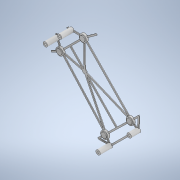
# Autodesk Inventor part: print006_Grundform_Boden
Saved by Autodesk Inventor 2020.3 (Build 243373000, 373)
## iProperties
Created: 2020-03-04
Part Number: print006_Grundform_Boden
Material: Generic
Document SubType Name: Modeling
Designer: Mara
Density: 1 g/cm^3
Appearance: Default
d0: 2,000 mm
d2: 1,000 mm
d3: 5,563 mm
d8: 5,563 mm
d9: 2,000 mm
d10: 170,74 deg
d11: 2,000 mm
d12: 163,54 deg
d21: 60,427 mm
d22: 66,844 mm
d24: 47,207 mm
d25: 2,000 mm
d26: 2,000 mm
d27: 81,43 deg
d28: 93,01 deg
d29: 53,219 mm
d30: 2,000 mm
d31: 2,000 mm
d32: 2,000 mm
d33: 2,000 mm
d34: 2,000 mm
d35: 2,000 mm
d36: 66,67 deg
d37: 45,78 deg
d39: 92,41 deg
d40: 87,65 deg
d42: 89,80 deg
d45: 1,000 mm
d46: 18,000 mm
d48: 2,000 mm
d49: 6,361 mm
d51: 27,126 mm
d52: 44,927 mm
d53: 48,903 mm
d54: 29,968 mm
d55: 20,958 mm
d56: 2,000 mm
d57: 2,000 mm
d58: 2,000 mm
d59: 64,660 mm
d60: 67,034 mm
d61: 34,990 mm
d62: 27,853 mm
d63: 15,000 mm
d64: 11,000 mm
d65: 20,850 mm
d66: 17,000 mm
d67: 11,000 mm
d70: 10,300 mm
d71: 3,845 mm
d72: 5,442 mm
d73: 5,436 mm
d75: 5,541 mm
d76: 5,457 mm
d77: 3,113 mm
d78: 2,630 mm
d80: 3,207 mm
d82: 5,463 mm
d87: 1,000 mm
d88: 0,00 deg
d93: 1,000 mm
d94: 4,757 mm
d95: 1,000 mm
d96: 4,757 mm
d99: 1,000 mm
d100: 4,757 mm
d105: 17,500 mm
d106: 1,000 mm
d107: 0,00 deg
d108: 0,00 deg
d109: 4,757 mm
d110: 1,000 mm
d111: 13,000 mm
d112: 1,000 mm
d113: 0,00 deg
d114: 0,00 deg
d115: 2,049 mm
d116: 2,049 mm
d117: 2,049 mm
d118: 3,300 mm
d119: 0,00 deg
d120: 2,049 mm
d121: 3,300 mm
d122: 0,00 deg
d123: 2,000 mm
d124: 0,00 deg
d125: 2,000 mm
d127: 2,000 mm
d128: 1,000 mm
d129: 0,00 deg
d130: 2,000 mm
d131: 2,000 mm
d134: 2,000 mm
d135: 2,000 mm
Author: Mara
Autodesk Inventor part; units mm, degrees
ref_plane "YZ Plane" through (0, 0, 0) normal (1, 0, 0) x (0, 1, 0)
ref_plane "XZ Plane" through (0, 0, 0) normal (0, 1, 0) x (-1, 0, 0)
ref_plane "XY Plane" through (0, 0, 0) normal (0, 0, 1) x (1, 0, 0)
sketch "Sketch1" plane through (0, 0, 0) normal (0, 0, 1) x (1, 0, 0)
  line L0 (-49.2977, 34.5359) -> (-22.38, 61.3045)
  line L1 (-47.8874, 33.1177) -> (-20.9698, 59.8864)
  line L2 (-49.2977, 34.5359) -> (-47.8874, 33.1177) construction
  circle A0 centre (-52.4729, 29.968) radius 5.563
  circle A1 centre (-17.7815, 64.4351) radius 5.563
  line L3 (-13.9364, 68.4553) -> (-0.1095, 78.3456)
  line L4 (-12.7631, 66.8356) -> (1.0638, 76.7259)
  line L5 (-57.711, 28.0946) -> (-67.3885, 22.8653)
  line L6 (-56.7093, 26.3625) -> (-66.3869, 21.1332)
  line L7 (-49.5894, 25.2106) -> (10.1162, -41.4966)
  circle A2 centre (14.4958, -44.9268) radius 5.563
  circle A3 centre (52.6405, -7.8239) radius 5.563
  line L8 (-48.0932, 26.5378) -> (11.6124, -40.1694)
  line L9 (-14.6001, 59.8716) -> (48.0505, -4.6808)
  line L10 (-13.1915, 61.292) -> (49.4591, -3.2604)
  line L11 (49.4227, -12.3618) -> (19.1106, -41.8201)
  line L12 (48.0258, -10.9306) -> (17.7136, -40.3888)
  line L13 (11.2885, -49.4721) -> (3.9093, -56.6581)
  line L14 (9.8883, -48.0441) -> (2.5091, -55.23)
  line L15 (57.2511, -4.7111) -> (65.1179, 2.9774)
  line L16 (55.8523, -3.2817) -> (63.7191, 4.4068)
  line L17 (-39.0119, 41.9442) -> (29.6903, -28.7495)
  line L18 (-37.5936, 43.3546) -> (31.1246, -27.3556)
  line L19 (-55.5021, 34.6339) -> (-60.6997, 47.8234)
  line L20 (-53.6558, 35.4038) -> (-59.1552, 49.3593)
  line L21 (-23.223, 65.5915) -> (-42.1516, 65.9031)
  line L22 (-23.2803, 63.5921) -> (-44.1303, 63.9354)
  circle A4 centre (-17.2221, 20.9576) radius 3.1804
  line L23 (13.0651, -39.5509) -> (-14.9644, 18.7175)
  line L24 (11.2563, -40.4044) -> (-16.7485, 17.8127)
  line L25 (-14.0533, 20.686) -> (47.9022, -4.9092)
  line L26 (-14.8421, 18.848) -> (47.1775, -6.7738)
  line L27 (-18.703, 58.9489) -> (-18.2564, 23.9652)
  line L28 (-16.7032, 58.9776) -> (-16.2565, 23.9879)
  line L29 (-47.4654, 27.5447) -> (-20.389, 20.6653)
  line L30 (-46.932, 29.4728) -> (-19.9371, 22.614)
  line L31 (-0.1095, 78.3456) -> (1.0638, 76.7259)
  line L32 (-44.073, 65.9347) -> (-44.1303, 63.9354) construction
  line L33 (-59.1552, 49.3593) -> (-61.0015, 48.5894) construction
  line L34 (-67.3885, 22.8653) -> (-66.3869, 21.1332)
  line L35 (3.9093, -56.6581) -> (2.5091, -55.23)
  line L36 (65.1179, 2.9774) -> (63.7191, 4.4068)
  line L37 (-59.1552, 49.3593) -> (-60.6997, 47.8234)
  line L38 (-44.1303, 63.9354) -> (-42.1516, 65.9031)
  line L39 (-42.1516, 65.9031) -> (-44.073, 65.9347) construction
  line L40 (-60.6997, 47.8234) -> (-61.0015, 48.5894) construction
  point P0 (0, 0)
  point P1 (9.143, -43.4122)
  point P2 (-19.963, 60.8956)
  point P3 (18.6755, -41.2556)
  point P4 (19.8991, -43.603)
  point P5 (47.2964, -9.3692)
  point P6 (58.0343, -9.1855)
  point P7 (55.8444, -3.2761)
  point P8 (16.2732, -50.1982)
  point P9 (18.0227, -49.2289)
  point P10 (56.2951, -12.0181)
  point P11 (57.5423, -10.4544)
  point P12 (-20.321, 22.7115)
  point P13 (-20.9757, 59.8805)
  point P14 (-18.6091, 23.8197)
  point P15 (10.5981, -39.0362)
  point P16 (31.0842, -30.1838)
  point P17 (32.5185, -28.7899)
  point P18 (31.1246, -27.3556)
  point P19 (-13.0632, 18.1131)
  point P20 (-13.5186, 15.7119)
  point P21 (29.6903, -28.7495)
  point P22 (-20.0433, 22.4258)
  dimension "d49" = 6.3609
  dimension "d0" = 2
  dimension "d2" = 1
  dimension "d3" = 5.563
  dimension "d8" = 5.563
  dimension "d9" = 2
  dimension "d10" = 170.735
  dimension "d11" = 2
  dimension "d12" = 163.544
  dimension "d21" = 60.4275
  dimension "d22" = 66.8436
  dimension "d24" = 47.2075
  dimension "d25" = 2
  dimension "d26" = 2
  dimension "d27" = 81.433
  dimension "d28" = 93.011
  dimension "d29" = 53.2188
  dimension "d30" = 2
  dimension "d31" = 2
  dimension "d32" = 2
  dimension "d33" = 2
  dimension "d34" = 2
  dimension "d35" = 2
  dimension "d36" = 66.667
  dimension "d37" = 45.784
  dimension "d39" = 92.41
  dimension "d40" = 87.648
  dimension "d42" = 89.8
  dimension "d45" = 1
  dimension "d46" = 18
  dimension "d48" = 2
  dimension "d51" = 27.126
  dimension "d52" = 44.9268
  dimension "d53" = 48.9027
  dimension "d54" = 29.968
  dimension "d55" = 20.9576
  dimension "d56" = 2
  dimension "d57" = 2
  dimension "d58" = 2
  dimension "d59" = 64.6596
  dimension "d60" = 67.0343
  dimension "d61" = 34.9897
  dimension "d62" = 27.8525
  dimension "d63" = 15
  dimension "d64" = 11
  dimension "d65" = 20.85
  dimension "d66" = 17
  dimension "d67" = 11
  dimension "d70" = 10.3
  dimension "d71" = 3.8451
  dimension "d72" = 5.4415
  dimension "d73" = 5.4358
  dimension "d75" = 5.5409
  dimension "d76" = 5.4575
  dimension "d77" = 3.1128
  dimension "d78" = 2.6305
  dimension "d80" = 3.2073
  dimension "d82" = 5.463
  constraints: 83 end point, 27 parallel, 4 point on line, 2 perpendicular, 62 other
  measures "d0" distance between parallel lines of L1 L0
  measures "d2" distance from line of L0 point (-52.473, 29.968)
  measures "d3" distance of L0.start point (-52.473, 29.968)
  measures "d8" distance of L0.end point (-17.782, 64.435)
  measures "d9" distance between parallel lines of L4 L3
  measures "d10" angle of L3 L0
  measures "d11" distance between parallel lines of L6 L5
  measures "d12" angle of L1 L6
  measures "d21" distance of point (-52.473, 29.968) point (0, 0)
  measures "d22" distance of point (0, 0) point (-17.782, 64.435)
  measures "d24" distance of point (0, 0) point (14.496, -44.927)
  measures "d25" distance between parallel lines of L7 L8
  measures "d26" distance between parallel lines of L9 L10
  measures "d27" angle of L10 L4
  measures "d28" angle of L8 L1
  measures "d29" distance of point (0, 0) point (52.641, -7.824)
  measures "d30" distance between parallel lines of L11 L12
  measures "d31" distance between parallel lines of L13 L14
  measures "d32" distance between parallel lines of L15 L16
  measures "d33" distance between parallel lines of L18 L17
  measures "d34" distance between parallel lines of L20 L19
  measures "d35" distance between parallel lines of L21 L22
  measures "d36" angle of L0 L20
  measures "d37" angle of L0 L22
  measures "d39" angle of L14 L7
  measures "d40" angle of L12 L8
  measures "d42" angle of L10 L16
  measures "d45" distance from line of point (-17.222, 20.958) L18
  measures "d46" distance from line of L17 point (-52.473, 29.968)
  measures "d48" distance between parallel lines of L23 L24
  measures "d51" distance of point (0, 0) point (-17.222, 20.958)
  measures "d52" vertical distance of point (0, 0) point (14.496, -44.927)
  measures "d53" distance of point (-52.473, 29.968) point (-17.782, 64.435)
  measures "d54" vertical distance of point (0, 0) point (-52.473, 29.968)
  measures "d55" vertical distance of point (-17.222, 20.958) point (0, 0)
  measures "d56" distance between parallel lines of L26 L25
  measures "d57" distance between parallel lines of L28 L27
  measures "d58" distance between parallel lines of L29 L30
  measures "d59" distance of L23.start L23.end
  measures "d60" distance of L25.start L25.end
  measures "d61" vertical distance of L28.start L28.end
  measures "d62" distance of L30.start L30.end
  measures "d63" distance of L20.start L20.end
  measures "d64" distance of L5.start L5.end
  measures "d65" horizontal distance of L22.start L22.end
  measures "d66" distance of L3.start L3.end
  measures "d67" distance of L15.start L15.end
  measures "d70" distance of L13.start L13.end
  measures "d71" horizontal distance of L3.start point (-17.782, 64.435)
  measures "d72" horizontal distance of point (-17.782, 64.435) L21.start
  measures "d73" vertical distance of point (-52.473, 29.968) L20.start
  measures "d75" horizontal distance of point (-52.473, 29.968) L30.start
  measures "d76" vertical distance of point (-17.782, 64.435) L28.start
  measures "d77" vertical distance of point (52.641, -7.824) L15.start
  measures "d78" vertical distance of point (52.641, -7.824) point (57.542, -10.454)
  measures "d80" horizontal distance of point (14.496, -44.927) L13.start
  measures "d82" horizontal distance of point (52.641, -7.824) L26.end
extrude "Extrusion3" add sketch "Sketch1" against normal blind 1 contours L0 A1 L1 A0 | A0 | A1 | A0 L19 L37 L20 | L22 L38 L21 A1 | L1 L18 A4 L30 L17 | A1 L28 A4 L27 | L17 A4 L29 A0 L30 | A0 L6 L34 L5 | L3 L31 L4 A1 | A4 L18 | L18 A4 L17 | L17 A4 | A4 L25 A3 L26 L18 | L18 L26 A4 | A1 L10 A3 L9 | A4 L23 L17 | L17 L23 A2 L8 L24 A4 | L8 L24 A2 L7 A0 | L18 L12 L17 L23 A4 L26 | A3 | L8 A2 L24 | A2 | L12 A3 L11 A2 | A2 L13 L35 L14 | L16 L36 L15 A3
sketch "Sketch3" plane through (0, 0, 0) normal (0, 0, 1) x (1, 0, 0)
  circle A0 centre (20.7546, -56.5669) radius 2.3783
  circle A1 centre (20.7546, -56.5669) radius 3.3783
  circle A2 centre (-36.8834, 64.7402) radius 2.3783
  circle A3 centre (-36.8834, 64.7402) radius 3.3783
  circle A4 centre (-58.3828, 44.2123) radius 2.3783
  circle A5 centre (-58.3828, 44.2123) radius 3.3783
  arc A6 (49.4227, -12.3618) -> (57.2511, -4.7111) centre (52.6405, -7.8239) ccw projected
  arc A7 (11.2885, -49.4721) -> (19.1106, -41.8201) centre (14.4958, -44.9268) ccw projected
  point P0 (0, 0)
  dimension "d93" = 1
  dimension "d94" = 4.7566
  dimension "d95" = 1
  dimension "d96" = 4.7566
  dimension "d99" = 1
  dimension "d100" = 4.7566
  constraints: 6 centre point, 3 coincident
  measures "d93" radial gap between concentric circles of A1 A0
  measures "d94" diameter of A0
  measures "d95" radial gap between concentric circles of A3 A2
  measures "d96" diameter of A2
  measures "d99" radial gap between concentric circles of A5 A4
  measures "d100" diameter of A4
extrude "Extrusion5" add sketch "Sketch3" along normal blind 17.5 and the other way blind 1
sketch "Sketch6" plane through (0, 0, 0) normal (0, 0, 1) x (1, 0, 0)
  circle A0 centre (62.8402, -15.6905) radius 2.3785
  circle A1 centre (62.8402, -15.6905) radius 3.3785
  point P0 (0, 0)
  dimension "d109" = 4.757
  dimension "d110" = 1
  constraints: 2 centre point, 1 coincident
  measures "d109" diameter of A0
  measures "d110" radial gap between concentric circles of A1 A0
extrude "Extrusion6" add sketch "Sketch6" along normal blind 13 and the other way blind 1
sketch "Sketch7" plane through (-58.3828, 44.2123, 17.5) normal (0, 0, 1) x (1, 0, 0)
  circle A0 centre (0, 0) radius 3.3783
  circle A1 centre (0, 0) radius 3.3783 projected
  circle A2 centre (0, 0) radius 1.3297
  circle A3 centre (21.4994, 20.5278) radius 3.3783
  circle A4 centre (21.4994, 20.5278) radius 3.3783 projected
  circle A5 centre (21.4994, 20.5278) radius 1.3293
  circle A6 centre (79.1375, -100.7793) radius 3.3783
  circle A7 centre (79.1375, -100.7793) radius 3.3783 projected
  circle A8 centre (79.1375, -100.7793) radius 1.3293
  point P0 (58.3828, -44.2123)
  dimension "d115" = 2.0486
  dimension "d116" = 2.049
  dimension "d117" = 2.049
  constraints: 6 centre point, 6 coincident, 3 concentric
  measures "d115" radial gap between concentric circles of A0 A2
  measures "d116" radial gap between concentric circles of A3 A5
  measures "d117" radial gap between concentric circles of A6 A8
extrude "Extrusion7" add sketch "Sketch7" against normal blind 3.3
sketch "Sketch8" plane through (62.8402, -15.6905, 13) normal (0, 0, 1) x (1, 0, 0)
  circle A0 centre (0, 0) radius 3.3785
  circle A1 centre (0, 0) radius 3.3785 projected
  circle A2 centre (0, 0) radius 1.3295
  point P0 (-62.8402, 15.6905)
  dimension "d120" = 2.049
  constraints: 2 centre point, 2 coincident, 1 concentric
  measures "d120" radial gap between concentric circles of A0 A2
extrude "Extrusion8" add sketch "Sketch8" against normal blind 3.3
sketch "Sketch9" plane through (0, 0, -1) normal (0, 0, -1) x (-1, 0, 0)
  circle A0 centre (58.3828, 44.2123) radius 2.3783
  arc A1 (58.0553, 46.568) -> (56.5363, 42.7134) centre (58.3828, 44.2123) ccw projected
  circle A2 centre (36.8834, 64.7402) radius 2.3783
  arc A3 (34.7075, 63.7802) -> (39.0899, 63.8524) centre (36.8834, 64.7402) ccw projected
  point P0 (0, 0)
  constraints: 2 centre point, 2 coincident, 2 concentric
extrude "Extrusion9" cut sketch "Sketch9" against normal blind 2
sketch "Sketch10" plane through (0, 0, 0) normal (0, 0, 1) x (1, 0, 0)
  arc A0 (49.4227, -12.3618) -> (57.2511, -4.7111) centre (52.6405, -7.8239) ccw projected
  line L0 (56.3201, -11.9961) -> (59.655, -14.5641)
  circle A1 centre (62.8402, -15.6905) radius 3.3785 projected
  line L1 (57.5579, -10.4251) -> (60.8502, -12.9602)
  arc A2 (11.2885, -49.4721) -> (19.1106, -41.8201) centre (14.4958, -44.9268) ccw projected
  line L2 (16.2829, -50.1949) -> (18.3621, -54.1818)
  circle A3 centre (20.7546, -56.5669) radius 3.3783 projected
  line L3 (18.0312, -49.2219) -> (20.1301, -53.2468)
  circle A4 centre (20.7546, -56.5669) radius 3.3783 projected
  arc A5 (11.2885, -49.4721) -> (19.1106, -41.8201) centre (14.4958, -44.9268) ccw projected
  line L4 (3.9093, -56.6581) -> (19.4284, -56.6581)
  circle A6 centre (20.7546, -56.5669) radius 1.3293 projected
  line L5 (3.9093, -56.6581) -> (11.2885, -49.4721) projected
  line L6 (5.9631, -54.6581) -> (17.9673, -54.6581)
  line L7 (65.1179, 2.9774) -> (64.168, -15.7578)
  circle A7 centre (62.8402, -15.6905) radius 1.3295 projected
  line L8 (65.1179, 2.9774) -> (57.2511, -4.7111) projected
  line L9 (63.0109, 0.9182) -> (62.3382, -12.3495)
  circle A8 centre (62.8402, -15.6905) radius 1.3295 projected
  line L10 (21.0962, -55.2822) -> (61.9032, -14.7472)
  line L11 (21.6812, -57.5201) -> (62.4982, -16.9752)
  circle A9 centre (-36.8834, 64.7402) radius 1.3293
  line L12 (-57.2083, 46.2804) -> (-39.1976, 64.1914)
  line L13 (-56.04, 44.6216) -> (-37.948, 62.6134)
  circle A10 centre (-36.8834, 64.7402) radius 2.3783 projected
  circle A11 centre (-58.3828, 44.2123) radius 2.3783 projected
  line L14 (-49.2977, 34.5359) -> (-22.38, 61.3045) projected
  point P0 (0, 0)
  point P1 (64.3253, -12.6559)
  point P2 (17.3775, -56.6581)
  point P3 (23.8949, -55.3212)
  point P4 (60.9635, -18.4998)
  point P5 (59.6997, -16.9361)
  point P6 (22.631, -53.7576)
  dimension "d125" = 2
  dimension "d127" = 2
  dimension "d130" = 2
  dimension "d131" = 2
  dimension "d134" = 2
  dimension "d135" = 2
  constraints: 24 end point, 18 point on circle, 7 parallel, 2 horizontal, 2 point on line, 1 centre point, 1 tangent, 5 other
  measures "d125" distance between parallel lines of L1 L0
  measures "d127" distance between parallel lines of L2 L3
  measures "d130" distance between parallel lines of L4 L6
  measures "d131" distance between parallel lines of L7 L9
  measures "d134" distance between parallel lines of L11 L10
  measures "d135" distance between parallel lines of L13 L12
extrude "Extrusion10" add sketch "Sketch10" against normal blind 1 contours A0 L1 A1 L0 | A1 L11 A3 L10 | L8 L7 A1 L9 | A3 L2 A2 L3 | L4 L5 L6 A3 | L12 A10 L13 A11
sketch "Sketch11" plane through (0, 0, 0) normal (0, 0, 1) x (1, 0, 0)
  circle A0 centre (-52.4729, 29.968) radius 5.563
  arc A1 (-49.2977, 34.5359) -> (-53.6558, 35.4038) centre (-52.4729, 29.968) ccw projected
  arc A2 (-56.7093, 26.3625) -> (-49.5894, 25.2106) centre (-52.4729, 29.968) ccw projected
  arc A3 (-55.5021, 34.6339) -> (-57.711, 28.0946) centre (-52.4729, 29.968) ccw projected
  circle A4 centre (-17.7815, 64.4351) radius 5.563
  circle A5 centre (14.4958, -44.9268) radius 5.563
  circle A6 centre (52.6405, -7.8239) radius 5.563
  point P0 (0, 0)
  point P1 (-13.9364, 68.4553)
  point P2 (-18.703, 58.9489)
  point P3 (-23.223, 65.5915)
  point P4 (17.7136, -40.3888)
  point P5 (11.2885, -49.4721)
  point P6 (10.1162, -41.4966)
  point P7 (55.8523, -3.2817)
  point P8 (56.3201, -11.9961)
  point P9 (47.1775, -6.7738)
  constraints: 11 point on circle, 4 centre point, 3 concentric
extrude "Extrusion11" add sketch "Sketch11" along normal blind 2
sketch "Sketch12" plane through (-52.4729, 29.968, 2) normal (0, 0, 1) x (1, 0, 0)
  circle A0 centre (0, 0) radius 3.9985
  circle A1 centre (0, 0) radius 5.563 projected
  circle A2 centre (34.6914, 34.4671) radius 5.563 projected
  circle A3 centre (34.6914, 34.4671) radius 3.9985
  circle A4 centre (66.9687, -74.8947) radius 5.563 projected
  circle A5 centre (66.9687, -74.8947) radius 3.9985
  circle A6 centre (105.1134, -37.7919) radius 5.563 projected
  circle A7 centre (105.1134, -37.7919) radius 3.9985
  point P0 (52.4729, -29.968)
  dimension "d138" = 7.997
  dimension "d139" = 1.5645
  dimension "d140" = 7.997
  dimension "d141" = 7.997
  dimension "d142" = 7.997
  constraints: 4 centre point, 3 coincident
  measures "d138" diameter of A0
  measures "d139" radial gap between concentric circles of A0 A1
  measures "d140" diameter of A3
  measures "d141" diameter of A5
  measures "d142" diameter of A7
extrude "Extrusion12" add sketch "Sketch12" along normal blind 1 contours A0 | A3 | A5 | A7
equation "\"d8\" = d3"
body "Solid1"
